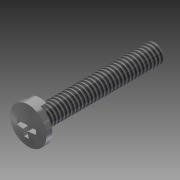
# Autodesk Inventor part: Prop Screw
Saved by Autodesk Inventor 2013 (Build 170138000, 138)
## iProperties
Created: 2014-08-02
Part Number: Prop Screw
Material: Stainless Steel
Document SubType Name: Modeling
Designer: Kyle
Density: 1 g/cm^3
Author: Kyle
Autodesk Inventor part; units mm, degrees
ref_plane "YZ Plane" through (0, 0, 0) normal (1, 0, 0) x (0, 1, 0)
ref_plane "XZ Plane" through (0, 0, 0) normal (0, 1, 0) x (-1, 0, 0)
sketch "Sketch1" plane through (0, 0, 0) normal (0, 0, 1) x (1, 0, 0)
  circle A0 centre (0, 0) radius 1.9685
  dimension "d0" = 3.937
  constraints: 1 centre point, 1 coincident
  measures "d0" diameter of A0
sketch "Sketch1 outline for Extrusion1" plane through (0, 0, 0) normal (0, 0, 1) x (1, 0, 0)
  circle A0 centre (0, 0) radius 1.9685
extrude "Extrusion1" add sketch "Sketch1 outline for Extrusion1" along normal blind 24.765
sketch "Sketch2" plane through (0, 0, 24.765) normal (0, 0, 1) x (1, 0, 0)
  circle A0 centre (0, 0) radius 1.9685
  line L0 (-1.397, 3.68081) -> (-1.397, 1.386861)
  line L1 (1.397, 3.68081) -> (1.397, 1.386861)
  line L2 (1.397, -3.68081) -> (1.397, -1.386861)
  line L3 (-1.397, -3.68081) -> (-1.397, -1.386861)
  arc A1 (1.397, 3.68081) -> (-1.397, 3.68081) centre (0, 0) ccw
  arc A2 (-1.397, -3.68081) -> (1.397, -3.68081) centre (0, 0) ccw
  arc A3 (-1.397, 1.386861) -> (-1.397, -1.386861) centre (0, 0) ccw
  arc A4 (1.397, -1.386861) -> (1.397, 1.386861) centre (0, 0) ccw
  point P0 (0, 1.9685)
  point P1 (0, -1.9685)
  point P2 (1.397, 1.9685)
  point P3 (-1.397, 1.9685)
  point P4 (1.397, -1.9685)
  point P5 (-1.397, -1.9685)
  dimension "d6" = 1.397
  dimension "d7" = 1.397
  dimension "d8" = 1.397
  dimension "d9" = 1.397
  constraints: 14 point on circle, 8 end point, 4 centre point, 3 equal length, 2 coincident, 1 vertical
  measures "d6" distance of point (1.397, 1.969) A0.start
  measures "d7" distance of point (-1.397, 1.969) A0.start
  measures "d8" distance of point (1.397, -1.969) A0.end
  measures "d9" distance of point (-1.397, -1.969) A0.end
sketch "Sketch2 outline for Extrusion2" plane through (0, 0, 24.765) normal (0, 0, 1) x (1, 0, 0)
  arc A0 (1.397, 3.68081) -> (-1.397, 3.68081) centre (0, 0) ccw
  line L0 (-1.397, 3.68081) -> (-1.397, 1.386861)
  arc A1 (-1.397, 1.386861) -> (-1.397, -1.386861) centre (0, 0) ccw
  line L1 (-1.397, -1.386861) -> (-1.397, -3.68081)
  arc A2 (-1.397, -3.68081) -> (1.397, -3.68081) centre (0, 0) ccw
  line L2 (1.397, -3.68081) -> (1.397, -1.386861)
  arc A3 (1.397, -1.386861) -> (1.397, 1.386861) centre (0, 0) ccw
  line L3 (1.397, 1.386861) -> (1.397, 3.68081)
extrude "Extrusion2" add sketch "Sketch2 outline for Extrusion2" along normal blind 1.27
sketch "Sketch3" plane through (0, 0, 26.035) normal (0, 0, 1) x (1, 0, 0)
  arc A0 (1.397, 3.68081) -> (-1.397, 3.68081) centre (0, 0) ccw
  circle A1 centre (0, 0) radius 3.937
  constraints: 1 centre point, 1 coincident
sketch "Sketch3 outline for Extrusion3" plane through (0, 0, 26.035) normal (0, 0, 1) x (1, 0, 0)
  circle A0 centre (0, 0) radius 3.937
extrude "Extrusion3" add sketch "Sketch3 outline for Extrusion3" along normal blind 1.27
ref_plane "Work Plane1" through (0, 0, 28.067) normal (0, 0, 1) x (1, 0, 0)
sketch "Sketch4" plane through (0, 0, 28.067) normal (0, 0, 1) x (1, 0, 0)
  circle A0 centre (0, 0) radius 0.127
  dimension "d15" = 0.254
  constraints: 1 centre point, 1 coincident
  measures "d15" diameter of A0
sketch "Sketch4 outline for Loft1" plane through (0, 0, 28.067) normal (0, 0, 1) x (1, 0, 0)
  circle A0 centre (0, 0) radius 0.127
loft "Loft1" add profiles "Sketch4 outline for Loft1" section 2 edges at (-3.937, 0, 27.305)
sketch "Sketch5" plane through (0, 0, 28.067) normal (0, 0, 1) x (1, 0, 0)
  circle A0 centre (0, 0) radius 0.127 projected
  line L0 (-0.508, 2.032) -> (0.508, 2.032)
  line L1 (0.508, 2.032) -> (0.508, 0.508)
  line L2 (0.508, 0.508) -> (2.032, 0.508)
  line L3 (2.032, 0.508) -> (2.032, -0.508)
  line L4 (2.032, -0.508) -> (0.508, -0.508)
  line L5 (0.508, -0.508) -> (0.508, -2.032)
  line L6 (0.508, -2.032) -> (-0.508, -2.032)
  line L7 (-0.508, -2.032) -> (-0.508, -0.508)
  line L8 (-0.508, -0.508) -> (-2.032, -0.508)
  line L9 (-2.032, -0.508) -> (-2.032, 0.508)
  line L10 (-2.032, 0.508) -> (-0.508, 0.508)
  line L11 (-0.508, 0.508) -> (-0.508, 2.032)
  dimension "d22" = 0.508
  dimension "d23" = 0.508
  dimension "d24" = 0.508
  dimension "d25" = 0.508
  dimension "d26" = 2.032
  dimension "d27" = 2.032
  dimension "d28" = 2.032
  dimension "d29" = 2.032
  dimension "d30" = 2.032
  dimension "d31" = 2.032
  dimension "d32" = 2.032
  dimension "d33" = 2.032
  constraints: 24 end point, 9 parallel, 1 collinear, 1 perpendicular
  measures "d22" horizontal distance of L1.end A0.centre
  measures "d23" horizontal distance of L1.end A0.centre
  measures "d24" horizontal distance of L7.end A0.centre
  measures "d25" horizontal distance of L7.end A0.centre
  measures "d26" horizontal distance of L2.end A0.centre
  measures "d27" horizontal distance of L3.end A0.centre
  measures "d28" vertical distance of L5.end A0.centre
  measures "d29" vertical distance of L6.end A0.centre
  measures "d30" horizontal distance of A0.centre L8.end
  measures "d31" horizontal distance of A0.centre L9.end
  measures "d32" vertical distance of A0.centre L0.start
  measures "d33" vertical distance of A0.centre L0.end
sketch "Sketch5 outline for Extrusion4" plane through (0, 0, 28.067) normal (0, 0, 1) x (1, 0, 0)
  line L0 (2.032, 0.508) -> (0.508, 0.508)
  line L1 (2.032, -0.508) -> (2.032, 0.508)
  line L2 (0.508, -0.508) -> (2.032, -0.508)
  line L3 (0.508, -2.032) -> (0.508, -0.508)
  line L4 (-0.508, -2.032) -> (0.508, -2.032)
  line L5 (-0.508, -0.508) -> (-0.508, -2.032)
  line L6 (-2.032, -0.508) -> (-0.508, -0.508)
  line L7 (-2.032, 0.508) -> (-2.032, -0.508)
  line L8 (-0.508, 0.508) -> (-2.032, 0.508)
  line L9 (-0.508, 2.032) -> (-0.508, 0.508)
  line L10 (0.508, 2.032) -> (-0.508, 2.032)
  line L11 (0.508, 0.508) -> (0.508, 2.032)
extrude "Extrusion4" cut sketch "Sketch5 outline for Extrusion4" against normal blind 1.27
thread "Thread1" size "6-32 UNC" class "2A" standard "ANSI Unified Screw Threads" full length
body "Solid1"
